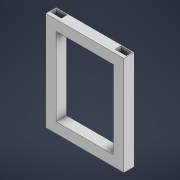
# Autodesk Inventor part: Shoulder_Cube_TestFit_V1
Saved by Autodesk Inventor 2022 (Build 260153000, 153)
## iProperties
Created: 2023-05-16
Part Number: Shoulder_Cube_TestFit_V1
Material: Generic
Document SubType Name: Modeling
Designer: Karl Spiteri
Density: 1 g/cm^3
Appearance: Default
Author: Karl Spiteri
Autodesk Inventor part; units mm, degrees
ref_plane "YZ Plane" through (0, 0, 0) normal (1, 0, 0) x (0, 1, 0)
ref_plane "XZ Plane" through (0, 0, 0) normal (0, 1, 0) x (-1, 0, 0)
ref_plane "XY Plane" through (0, 0, 0) normal (0, 0, 1) x (1, 0, 0)
sketch "Sketch1" plane through (0, 0, 0) normal (0, 0, 1) x (1, 0, 0)
  line L0 (0, 0) -> (-75, 0)
  line L1 (-75, 0) -> (-75, 95)
  line L2 (-75, 95) -> (0, 95)
  line L3 (0, 95) -> (0, 0)
  line L4 (-65, 85) -> (-10, 85)
  line L5 (-10, 85) -> (-10, 10)
  line L6 (-10, 10) -> (-65, 10)
  line L7 (-65, 10) -> (-65, 85)
  dimension "d0" = 75
  dimension "d1" = 95
  dimension "d10" = 55
  dimension "d11" = 75
  constraints: 16 end point, 4 parallel, 2 horizontal, 2 perpendicular
  measures "d0" distance of L1.end L2.end
  measures "d1" distance of L0.end L1.end
  measures "d10" distance of L5.end L6.end
  measures "d11" distance of L4.end L5.end
extrude "Extrusion3" add sketch "Sketch1" along normal blind 10
sketch "Sketch2" plane through (-75, 95, 0) normal (0, 1, 0) x (1, 0, 0)
  line L0 (1, -1) -> (11.6, -1)
  line L1 (11.6, -1) -> (11.6, -6.6)
  line L2 (11.6, -6.6) -> (1, -6.6)
  line L3 (1, -6.6) -> (1, -1)
  line L4 (74, -1) -> (63.4, -1)
  line L5 (63.4, -1) -> (63.4, -6.6)
  line L6 (63.4, -6.6) -> (74, -6.6)
  line L7 (74, -6.6) -> (74, -1)
  point P0 (75, 0)
  dimension "d14" = 10.6
  dimension "d15" = 5.6
  dimension "d16" = 10.6
  dimension "d17" = 5.6
  constraints: 16 end point, 4 parallel, 2 horizontal, 2 perpendicular
  measures "d14" distance of L1.end L2.end
  measures "d15" distance of L0.end L1.end
  measures "d16" distance of L6.end L5.end
  measures "d17" distance of L5.end L4.end
extrude "Extrusion4" cut sketch "Sketch2" against normal blind 5
sketch "Sketch3" plane through (-75, 0, 0) normal (0, -1, 0) x (1, 0, 0)
  line L0 (1, 1) -> (11.6, 1)
  line L1 (11.6, 1) -> (11.6, 6.6)
  line L2 (11.6, 6.6) -> (1, 6.6)
  line L3 (1, 6.6) -> (1, 1)
  line L4 (63.4, 6.6) -> (63.4, 1) projected
  line L5 (74, 1) -> (63.4, 1)
  line L6 (63.4, 1) -> (63.4, 6.6)
  line L7 (63.4, 6.6) -> (74, 6.6)
  line L8 (74, 6.6) -> (74, 1)
  point P0 (75, 0)
  point P1 (63.4, 1)
  dimension "d20" = 10.6
  dimension "d21" = 5.6
  dimension "d22" = 10.6
  dimension "d23" = 5.6
  constraints: 16 end point, 4 parallel, 2 horizontal, 2 perpendicular
  measures "d20" distance of L2.end L1.end
  measures "d21" distance of L1.end L0.end
  measures "d22" distance of L4.start L7.end
  measures "d23" distance of L5.end L4.start
extrude "Extrusion5" cut sketch "Sketch3" against normal blind 5
body "Solid3"
